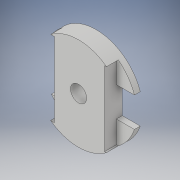
# Autodesk Inventor part: fakebattergasket3
Saved by Autodesk Inventor 2018.3 (Build 223284000, 284)
## iProperties
Created: 2019-09-05
Part Number: fakebattergasket3
Material: Generic
Document SubType Name: Modeling
Designer: Srinity
Density: 1 g/cm^3
Appearance: Default
Author: Srinity
Autodesk Inventor part; units mm, degrees
ref_plane "YZ Plane" through (0, 0, 0) normal (1, 0, 0) x (0, 1, 0)
ref_plane "XZ Plane" through (0, 0, 0) normal (0, 1, 0) x (-1, 0, 0)
ref_plane "XY Plane" through (0, 0, 0) normal (0, 0, 1) x (1, 0, 0)
sketch "Sketch1" plane through (0, 0, 0) normal (0, 0, 1) x (1, 0, 0)
  circle A0 centre (0, 0) radius 15.875
  circle A1 centre (0, 0) radius 2.75
  dimension "d0" = 31.75
  dimension "d1" = 5.5
  constraints: 2 centre point, 2 coincident
  measures "d0" diameter of A0
  measures "d1" diameter of A1
extrude "Extrusion1" add sketch "Sketch1" along normal blind 6
sketch "Sketch2" plane through (0, 0, 6) normal (0, 0, 1) x (1, 0, 0)
  line L0 (-17.145, 8.763) -> (-8.255, 8.763)
  line L1 (-8.255, 8.763) -> (-8.255, -8.763)
  line L2 (-8.255, -8.763) -> (-17.145, -8.763)
  line L3 (-17.145, -8.763) -> (-17.145, 8.763)
  line L4 (8.89, 5.08) -> (16.51, 5.08)
  line L5 (16.51, 5.08) -> (16.51, -5.08)
  line L6 (16.51, -5.08) -> (8.89, -5.08)
  line L7 (8.89, -5.08) -> (8.89, 5.08)
  line L8 (-12.7, 8.763) -> (-12.7, -8.763) construction
  line L9 (12.7, 5.08) -> (12.7, -5.08) construction
  point P0 (0, 0)
  point P1 (-8.255, 0)
  point P2 (8.89, 0)
  dimension "d4" = 8.89
  dimension "d5" = 7.62
  dimension "d6" = 10.16
  dimension "d7" = 12.7
  dimension "d8" = 12.7
  dimension "d9" = 17.526
  constraints: 20 end point, 6 midpoint, 4 parallel, 2 horizontal, 2 horizontal alignment, 2 perpendicular
  measures "d4" distance of L0.start L0.end
  measures "d5" distance of L4.start L4.end
  measures "d6" distance of L6.end L4.start
  measures "d7" distance from line of point (0, 0) L8
  measures "d8" distance from line of L9 point (0, 0)
  measures "d9" distance of L2.end L0.start
extrude "Extrusion2" cut sketch "Sketch2" against normal through all
sketch "Sketch3" plane through (0, 0, 6) normal (0, 0, 1) x (1, 0, 0)
  line L0 (-21.6805, 12.7) -> (-8.255, 12.7)
  line L1 (-8.255, 12.7) -> (-8.255, -12.7)
  line L2 (-8.255, -12.7) -> (-21.6805, -12.7)
  line L3 (-21.6805, -12.7) -> (-21.6805, 12.7)
  line L4 (-8.255, 8.763) -> (-8.255, -8.763) projected
  line L5 (8.89, 12.7) -> (29.1291, 12.7)
  line L6 (29.1291, 12.7) -> (29.1291, -12.7)
  line L7 (29.1291, -12.7) -> (8.89, -12.7)
  line L8 (8.89, -12.7) -> (8.89, 12.7)
  line L9 (8.89, -5.08) -> (8.89, 5.08) projected
  point P0 (0, 0)
  point P1 (-21.6805, 0)
  dimension "d12" = 25.4
  constraints: 16 end point, 4 collinear, 4 parallel, 2 horizontal, 2 perpendicular, 1 horizontal alignment, 1 midpoint
  measures "d12" distance of L2.end L0.start
extrude "Extrusion3" cut sketch "Sketch3" against normal blind 4
equation "\"d8\" = d7"
body "Solid1"
